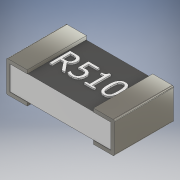
# Autodesk Inventor part: 21-1001
Saved by Autodesk Inventor 2018 (Build 220112000, 112)
## iProperties
Created: 2019-09-21
Part Number: 21-1001
Material: Copper
Document SubType Name: Modeling
Designer: Bradley
Density: 8.94 g/cm^3
Appearance: Smooth - White
Author: Bradley
Autodesk Inventor part; units mm, degrees
ref_plane "YZ Plane" through (0, 0, 0) normal (1, 0, 0) x (0, 1, 0)
ref_plane "XZ Plane" through (0, 0, 0) normal (0, 1, 0) x (-1, 0, 0)
ref_plane "XY Plane" through (0, 0, 0) normal (0, 0, 1) x (1, 0, 0)
sketch "Sketch1" plane through (0, 0, 0) normal (0, 1, 0) x (-1, 0, 0)
  line L0 (0.725, 0.175) -> (-0.725, 0.175)
  line L1 (-0.725, 0.175) -> (-0.725, -0.175)
  line L2 (-0.725, -0.175) -> (0.725, -0.175)
  line L3 (0.725, -0.175) -> (0.725, 0.175)
  line L4 (0.475, 0.175) -> (0.475, 0.225)
  line L5 (0.475, 0.225) -> (0.775, 0.225)
  line L6 (0.775, 0.225) -> (0.775, -0.225)
  line L7 (0.775, -0.225) -> (0.475, -0.225)
  line L8 (0.475, -0.225) -> (0.475, -0.175)
  line L9 (-0.475, 0.175) -> (-0.475, 0.225)
  line L10 (-0.475, 0.225) -> (-0.775, 0.225)
  line L11 (-0.775, 0.225) -> (-0.775, -0.225)
  line L12 (-0.775, -0.225) -> (-0.475, -0.225)
  line L13 (-0.475, -0.175) -> (-0.475, -0.225)
  line L14 (0.475, 0.175) -> (-0.475, 0.175)
  point P0 (0, 0)
  point P1 (0, 0.175)
  point P2 (0.725, 0)
  dimension "d0" = 1.55
  dimension "d1" = 0.05
  dimension "d2" = 0.05
  dimension "d3" = 0.45
  dimension "d4" = 0.3
  constraints: 30 end point, 12 point on line, 7 perpendicular, 3 collinear, 3 midpoint, 2 parallel, 1 horizontal, 1 horizontal alignment, 1 vertical, 1 vertical alignment
  measures "d0" distance between parallel lines of L11 L6
  measures "d1" distance of L7.end L8.end
  measures "d2" distance between parallel lines of L6 L3
  measures "d3" distance of L5.end L6.end
  measures "d4" distance of L6.end L7.end
extrude "Extrusion1" add sketch "Sketch1" along normal mid plane 0.85 contours L0 L4 L5 L6 L7 L8 L2 L3 | L0 L1 L2 L13 L12 L11 L10 L9
extrude "Extrusion2" add sketch "Sketch1" along normal mid plane 0.84 contours L3 L2 L1 L0
sketch "Sketch2" plane through (-0.475, -0.42, 0.175) normal (0, 0, 1) x (1, 0, 0)
  line L0 (0, 0) -> (0, 0.84) projected
  line L1 (0.95, 0) -> (0, 0) projected
  line L2 (0.95, 0) -> (0.95, 0.84) projected
  line L3 (0, 0.84) -> (0.95, 0.84) projected
  line L4 (0, 0.42) -> (0.95, 0.42) construction
  line L5 (0.2719, 0.27) -> (0.2201, 0.27)
  line L6 (0.2201, 0.27) -> (0.1253, 0.3894)
  line L7 (0.1253, 0.3894) -> (0.0796, 0.3894)
  line L8 (0.0796, 0.3894) -> (0.0796, 0.27)
  line L9 (0.0796, 0.27) -> (0.0397, 0.27)
  line L10 (0.0397, 0.27) -> (0.0397, 0.57)
  line L11 (0.0397, 0.57) -> (0.117, 0.57)
  spline S0 degree 2 poles (0.117, 0.57) (0.1428, 0.57) (0.1776, 0.5644) (0.1934, 0.5542) knots 0 0 0 1 2 2 2
  spline S1 degree 2 poles (0.1934, 0.5542) (0.2092, 0.544) (0.2274, 0.5121) (0.2274, 0.4886) knots 0 0 0 1 2 2 2
  spline S2 degree 2 poles (0.2274, 0.4886) (0.2274, 0.4557) (0.1938, 0.4112) (0.1652, 0.4006) knots 0 0 0 1 2 2 2
  line L12 (0.1652, 0.4006) -> (0.2719, 0.27)
  spline S3 degree 2 poles (0.1858, 0.4854) (0.1858, 0.4985) (0.1766, 0.5187) (0.1669, 0.5253) knots 0 0 0 1 2 2 2
  spline S4 degree 2 poles (0.1669, 0.5253) (0.1583, 0.5309) (0.1357, 0.5355) (0.1192, 0.5355) knots 0 0 0 1 2 2 2
  line L13 (0.1192, 0.5355) -> (0.0796, 0.5355)
  line L14 (0.0796, 0.5355) -> (0.0796, 0.4227)
  line L15 (0.0796, 0.4227) -> (0.1146, 0.4227)
  spline S5 degree 2 poles (0.1146, 0.4227) (0.1318, 0.4227) (0.1593, 0.4288) (0.1688, 0.4382) knots 0 0 0 1 2 2 2
  spline S6 degree 2 poles (0.1688, 0.4382) (0.1776, 0.4465) (0.1858, 0.4698) (0.1858, 0.4854) knots 0 0 0 1 2 2 2
  spline S7 degree 2 poles (0.469, 0.3653) (0.469, 0.3437) (0.4552, 0.3067) (0.4425, 0.2931) knots 0 0 0 1 2 2 2
  spline S8 degree 2 poles (0.4425, 0.2931) (0.4299, 0.2795) (0.3922, 0.2637) (0.3689, 0.2637) knots 0 0 0 1 2 2 2
  spline S9 degree 2 poles (0.3689, 0.2637) (0.3475, 0.2637) (0.3057, 0.2732) (0.2904, 0.2807) knots 0 0 0 1 2 2 2
  line L16 (0.2904, 0.2807) -> (0.2904, 0.3232)
  line L17 (0.2904, 0.3232) -> (0.2933, 0.3232)
  spline S10 degree 2 poles (0.2933, 0.3232) (0.2979, 0.3198) (0.3152, 0.3111) (0.3256, 0.3072) knots 0 0 0 1 2 2 2
  spline S11 degree 2 poles (0.3256, 0.3072) (0.3375, 0.3031) (0.3572, 0.2984) (0.3696, 0.2984) knots 0 0 0 1 2 2 2
  spline S12 degree 2 poles (0.3696, 0.2984) (0.3818, 0.2984) (0.4046, 0.3072) (0.4129, 0.3167) knots 0 0 0 1 2 2 2
  spline S13 degree 2 poles (0.4129, 0.3167) (0.4204, 0.3257) (0.4282, 0.3495) (0.4282, 0.3655) knots 0 0 0 1 2 2 2
  spline S14 degree 2 poles (0.4282, 0.3655) (0.4282, 0.3816) (0.4194, 0.402) (0.4112, 0.4088) knots 0 0 0 1 2 2 2
  spline S15 degree 2 poles (0.4112, 0.4088) (0.4027, 0.4164) (0.3774, 0.4227) (0.3621, 0.4227) knots 0 0 0 1 2 2 2
  spline S16 degree 2 poles (0.3621, 0.4227) (0.3455, 0.4227) (0.3127, 0.4176) (0.3028, 0.4154) knots 0 0 0 1 2 2 2
  line L18 (0.3028, 0.4154) -> (0.3028, 0.57)
  line L19 (0.3028, 0.57) -> (0.4673, 0.57)
  line L20 (0.4673, 0.57) -> (0.4673, 0.5347)
  line L21 (0.4673, 0.5347) -> (0.3414, 0.5347)
  line L22 (0.3414, 0.5347) -> (0.3414, 0.4548)
  spline S17 degree 2 poles (0.3414, 0.4548) (0.3487, 0.4557) (0.3628, 0.4565) (0.3686, 0.4565) knots 0 0 0 1 2 2 2
  spline S18 degree 2 poles (0.3686, 0.4565) (0.3917, 0.4565) (0.4236, 0.4489) (0.4382, 0.4377) knots 0 0 0 1 2 2 2
  spline S19 degree 2 poles (0.4382, 0.4377) (0.453, 0.4266) (0.469, 0.3925) (0.469, 0.3653) knots 0 0 0 1 2 2 2
  line L23 (0.6823, 0.27) -> (0.5359, 0.27)
  line L24 (0.5359, 0.27) -> (0.5359, 0.3006)
  line L25 (0.5359, 0.3006) -> (0.5904, 0.3006)
  line L26 (0.5904, 0.3006) -> (0.5904, 0.5017)
  line L27 (0.5904, 0.5017) -> (0.5359, 0.5017)
  line L28 (0.5359, 0.5017) -> (0.5359, 0.5292)
  spline S20 degree 2 poles (0.5359, 0.5292) (0.5668, 0.5292) (0.5959, 0.5467) (0.5979, 0.571) knots 0 0 0 1 2 2 2
  line L29 (0.5979, 0.571) -> (0.629, 0.571)
  line L30 (0.629, 0.571) -> (0.629, 0.3006)
  line L31 (0.629, 0.3006) -> (0.6823, 0.3006)
  line L32 (0.6823, 0.3006) -> (0.6823, 0.27)
  spline S21 degree 2 poles (0.9241, 0.42) (0.9241, 0.3393) (0.8772, 0.2637) (0.8284, 0.2637) knots 0 0 0 1 2 2 2
  spline S22 degree 2 poles (0.8284, 0.2637) (0.7788, 0.2637) (0.7323, 0.3407) (0.7323, 0.4198) knots 0 0 0 1 2 2 2
  spline S23 degree 2 poles (0.7323, 0.4198) (0.7323, 0.501) (0.7793, 0.5761) (0.8284, 0.5761) knots 0 0 0 1 2 2 2
  spline S24 degree 2 poles (0.8284, 0.5761) (0.8777, 0.5761) (0.9241, 0.4983) (0.9241, 0.42) knots 0 0 0 1 2 2 2
  spline S25 degree 2 poles (0.8726, 0.3286) (0.8784, 0.3434) (0.8833, 0.3891) (0.8833, 0.42) knots 0 0 0 1 2 2 2
  spline S26 degree 2 poles (0.8833, 0.42) (0.8833, 0.4509) (0.8784, 0.4963) (0.8724, 0.5117) knots 0 0 0 1 2 2 2
  spline S27 degree 2 poles (0.8724, 0.5117) (0.8663, 0.527) (0.8451, 0.5428) (0.8284, 0.5428) knots 0 0 0 1 2 2 2
  spline S28 degree 2 poles (0.8284, 0.5428) (0.8116, 0.5428) (0.79, 0.527) (0.7836, 0.5112) knots 0 0 0 1 2 2 2
  spline S29 degree 2 poles (0.7836, 0.5112) (0.7776, 0.4959) (0.7732, 0.4492) (0.7732, 0.4198) knots 0 0 0 1 2 2 2
  spline S30 degree 2 poles (0.7732, 0.4198) (0.7732, 0.3882) (0.7771, 0.3459) (0.7834, 0.3293) knots 0 0 0 1 2 2 2
  spline S31 degree 2 poles (0.7834, 0.3293) (0.7892, 0.3138) (0.8109, 0.297) (0.8284, 0.297) knots 0 0 0 1 2 2 2
  spline S32 degree 2 poles (0.8284, 0.297) (0.8449, 0.297) (0.8665, 0.3128) (0.8726, 0.3286) knots 0 0 0 1 2 2 2
  point P0 (0.475, 0.42)
  constraints: 2 end point, 2 midpoint, 1 horizontal
extrude "Extrusion3" add sketch "Sketch2" along normal blind 0.02 contours L5 L6 L7 L8 L9 L10 L11 S0 S1 S2 L12 | S7 S8 S9 L16 L17 S10 S11 S12 S13 S14 S15 S16 L18 L19 L20 L21 L22 S17 S18 S19 | L23 L24 L25 L26 L27 L28 S20 L29 L30 L31 L32 | S21 S22 S23 S24
fillet "Fillet1" radius 0.02 4 edges at (-0.775, 0, 0.225) (-0.775, 0, -0.225) (0.775, 0, 0.225) (0.775, 0, -0.225)
equation "\"d2\" = d1"
body "Solid1"
